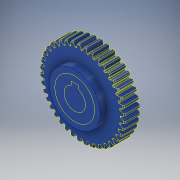
# Autodesk Inventor part: gear1
Saved by Autodesk Inventor 2018 (Build 220112000, 112)
## iProperties
Created: 2019-02-16
Part Number: gear1
Material: Generic
Description: SolidWorks IGES file using analytic representation for surfaces
Document SubType Name: Modeling
Designer: snipe
Density: 1 g/cm^3
Appearance: Blue - Wall Paint - Glossy
Sending System: SolidWorks 2018
Preprocessor: SolidWorks 2018
Minimum Resolution: 0.0
Sending System Product ID: 48_gear1
Receiving System Product ID: 48_gear1
Sent Units: Millimeter
Translation Standard: IGES 5.3
Model Creation Time: 2019-02-16
Title: C:\Users\Admin\Desktop\48_gear1.IGS
Author: Admin
Autodesk Inventor part; units mm, degrees
ref_plane "YZ Plane" through (0, 0, 0) normal (1, 0, 0) x (0, 1, 0)
ref_plane "XZ Plane" through (0, 0, 0) normal (0, 1, 0) x (-1, 0, 0)
ref_plane "XY Plane" through (0, 0, 0) normal (0, 0, 1) x (1, 0, 0)
surface "Composite1"
sketch "Sketch1" plane through (0, 0, 15) normal (0, 0, 1) x (1, 0, 0)
  circle A0 centre (0, 0) radius 25
  constraints: 1 centre point
extrude "Extrusion1" add sketch "Sketch1" against normal up to surface (30 mm away)
body "Solid1"
body "Srf1"
